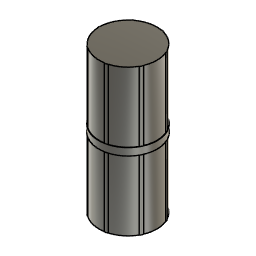
GYRO-MOUSE v19 (Autodesk Fusion 360 archive; units mm, degrees)
design "GYRO-MOUSE PART7"
Autodesk Fusion 360 part; units mm, degrees
sketch "Schizzo6" plane through (0, 0, 0) normal (0, 0, 1) x (1, 0, 0)
  circle A0 centre (0, 0) radius 3.95
  dimension "d41" = 7.9
  constraint coincident A0.centre origin
  measures "d41" diameter of A0
extrude "Estrusione5" add sketch "Schizzo6" along normal blind 20
sketch "Schizzo7" plane through (0, 0, 20) normal (0, 0, 1) x (-1, 0, 0)
  circle A0 centre (0, 0) radius 3.95
  circle A1 centre (3.5, 0) radius 0.5
  line L0 (0, 0) -> (3.5, 0)
  dimension "d44" = 1
  dimension "d45" = 3.5
  constraint coincident A0.centre L0.start
  constraint horizontal L0
  constraint coincident A1.centre L0.end
  measures "d44" diameter of A1
  measures "d45" distance of A0.centre A1.centre
extrude "Estrusione6" add sketch "Schizzo7" against normal up to surface (20 mm away) contours A0 A1 picked at (3.9652, 0.0457)
pattern_circular "Serie C1" count 7 over 360 about axis through (0, 0, 0) along (0, 0, 1) of "Estrusione6"
ref_plane "Piano di lavoro1" through (0.1035, 0, 10) normal (0, 0, 1) x (1, 0, 0)
sketch "Schizzo8" plane through (0, 0, 10) normal (0, 0, 1) x (1, 0, 0)
  circle A0 centre (0, 0) radius 4
  dimension "d50" = 8
  constraint coincident A0.centre origin
  measures "d50" diameter of A0
extrude "Estrusione7" add sketch "Schizzo8" along normal mid plane 1
equation "d45 = ( ( 8 - 1 ) / 2 ) * 1 mm"

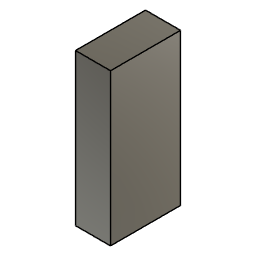
design "GYRO-MOUSE PART3"
Autodesk Fusion 360 part; units mm, degrees
sketch "Schizzo1" plane through (0, 0, 0) normal (0, 0, 1) x (1, 0, 0)
  line L0 (-1.5, 0) -> (1.5, 0)
  line L1 (1.5, 0) -> (1.5, 6)
  line L2 (1.5, 6) -> (-1.5, 6)
  line L3 (-1.5, 6) -> (-1.5, 0)
  dimension "d1" = 6
  dimension "d2" = 3
  constraint horizontal L0
  constraint vertical L1
  constraint horizontal L2
  constraint vertical L3
  constraint midpoint origin L0
  measures "d1" distance of L0.start L2.end
  measures "d2" distance of L1.end L2.end
extrude "Estrusione1" add sketch "Schizzo1" along normal blind 13
